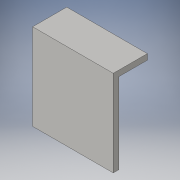
# Autodesk Inventor part: CapLiftHolder
Saved by Autodesk Inventor 2016 (Build 200138000, 138)
## iProperties
Created: 2017-01-28
Part Number: CapLiftHolder
Material: Generic
Document SubType Name: Modeling
Designer: RoboticsUser
Density: 1 g/cm^3
Appearance: Default
Mass: 0.58615 g
Surface Area: 10.3391 cm^2
Volume: 0.58615 cm^3
Author: RoboticsUser
Autodesk Inventor part; units mm, degrees
ref_plane "YZ Plane" through (0, 0, 0) normal (1, 0, 0) x (0, 1, 0)
ref_plane "XZ Plane" through (0, 0, 0) normal (0, 1, 0) x (-1, 0, 0)
ref_plane "XY Plane" through (0, 0, 0) normal (0, 0, 1) x (1, 0, 0)
sketch "Sketch1" plane through (0, 0, 0) normal (0, 0, 1) x (1, 0, 0)
  line L0 (0, 0) -> (18.0086, 0)
  line L1 (18.0086, 0) -> (18.0086, 18.0086)
  line L2 (18.0086, 18.0086) -> (0, 18.0086)
  line L3 (0, 18.0086) -> (0, 0)
  dimension "d0" = 18.0086
  dimension "d1" = 18.0086
  constraints: 8 end point, 2 parallel, 1 horizontal, 1 perpendicular
  measures "d0" distance of L2.end L1.end
  measures "d1" distance of L1.end L0.end
extrude "Extrusion1" add sketch "Sketch1" along normal blind 1.27
sketch "Sketch2" plane through (0, 18.0086, 0) normal (0, 1, 0) x (1, 0, 0)
  line L0 (0, 0) -> (18.0086, 0)
  line L1 (18.0086, 0) -> (18.0086, 6.35)
  line L2 (18.0086, 6.35) -> (0, 6.35)
  line L3 (0, 6.35) -> (0, 0)
  dimension "d4" = 6.35
  constraints: 8 end point, 2 parallel, 1 horizontal, 1 perpendicular
  measures "d4" distance of L1.end L0.end
extrude "Extrusion2" add sketch "Sketch2" along normal blind 1.27
sketch "Sketch3" plane through (0, 18.0086, 1.27) normal (0, 1, 0) x (1, 0, 0)
  line L0 (18.0086, 0) -> (0, 0) projected
  line L1 (0, 0) -> (18.0086, 0)
  line L2 (18.0086, 0) -> (18.0086, 1.27)
  line L3 (18.0086, 1.27) -> (0, 1.27)
  line L4 (0, 1.27) -> (0, 0)
  point P0 (0, 1.27)
  constraints: 8 end point, 2 parallel, 1 horizontal, 1 perpendicular
extrude "Extrusion3" add sketch "Sketch3" along normal blind 1.27
body "Solid1"
